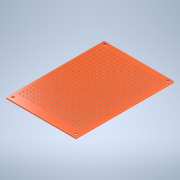
# Autodesk Inventor part: podložka na arduino
Saved by Autodesk Inventor 2022 (Build 260153000, 153)
## iProperties
Created: 2022-02-10
Part Number: podložka na arduino
Material: Generic
Document SubType Name: Modeling
Designer: matys
Density: 1 g/cm^3
Appearance: Smooth - Light Orange
Author: matys
Autodesk Inventor part; units mm, degrees
ref_plane "YZ Plane" through (0, 0, 0) normal (1, 0, 0) x (0, 1, 0)
ref_plane "XZ Plane" through (0, 0, 0) normal (0, 1, 0) x (-1, 0, 0)
ref_plane "XY Plane" through (0, 0, 0) normal (0, 0, 1) x (1, 0, 0)
sketch "Sketch1" plane through (0, 0, 0) normal (0, 1, 0) x (-1, 0, 0)
  line L0 (0, 0) -> (0, -70)
  line L1 (0, -70) -> (50, -70)
  line L2 (50, -70) -> (50, 0)
  line L3 (50, 0) -> (0, 0)
  dimension "d0" = 70
  dimension "d1" = 50
  constraints: 8 end point, 3 perpendicular, 1 vertical
  measures "d0" distance of L0.start L0.end
  measures "d1" distance of L0.end L1.end
extrude "Extrusion1" add sketch "Sketch1" along normal blind 1
sketch "Sketch2" plane through (0, 1, 0) normal (0, 1, 0) x (1, 0, 0)
  line L0 (0, 70) -> (-50, 70) projected
  line L1 (-50, 70) -> (-50, 68)
  line L2 (-50, 70) -> (-50, 0) projected
  line L3 (-50, 68) -> (-47.5, 68)
  line L4 (-47.5, 68) -> (-47.5, 70)
  line L5 (-47.5, 70) -> (-50, 70)
  line L6 (-50, 70) -> (0, 70)
  line L7 (0, 70) -> (-25, 70)
  line L8 (-25, 70) -> (-25, 0)
  line L9 (-25, 0) -> (-25, 70)
  circle A0 centre (-47.5, 68) radius 1
  circle A1 centre (-2.5, 68) radius 1
  line L10 (-50, 0) -> (-50, 2.5)
  line L11 (-50, 2.5) -> (-47.5, 2.5)
  line L12 (-47.5, 2.5) -> (-47.5, 0)
  line L13 (-50, 0) -> (0, 0) projected
  circle A2 centre (-47.5, 2.5) radius 1
  circle A3 centre (-2.5, 2.5) radius 1
  line L14 (-50, 70) -> (-47, 70)
  line L15 (-47, 70) -> (-47, 64.5)
  line L16 (-47, 64.5) -> (-50, 64.5)
  circle A4 centre (-47, 64.5) radius 0.5
  circle A5 centre (-47, 62) radius 0.5
  circle A6 centre (-47, 59.5) radius 0.5
  circle A7 centre (-47, 57) radius 0.5
  circle A8 centre (-47, 54.5) radius 0.5
  circle A9 centre (-47, 52) radius 0.5
  circle A10 centre (-47, 49.5) radius 0.5
  circle A11 centre (-47, 47) radius 0.5
  circle A12 centre (-47, 44.5) radius 0.5
  circle A13 centre (-47, 42) radius 0.5
  circle A14 centre (-47, 39.5) radius 0.5
  circle A15 centre (-47, 37) radius 0.5
  circle A16 centre (-47, 34.5) radius 0.5
  circle A17 centre (-47, 32) radius 0.5
  circle A18 centre (-47, 29.5) radius 0.5
  circle A19 centre (-47, 27) radius 0.5
  circle A20 centre (-47, 24.5) radius 0.5
  circle A21 centre (-47, 22) radius 0.5
  circle A22 centre (-47, 19.5) radius 0.5
  circle A23 centre (-47, 17) radius 0.5
  circle A24 centre (-47, 14.5) radius 0.5
  circle A25 centre (-47, 12) radius 0.5
  circle A26 centre (-47, 9.5) radius 0.5
  circle A27 centre (-47, 7) radius 0.5
  circle A28 centre (-44.5, 64.5) radius 0.5
  circle A29 centre (-44.5, 62) radius 0.5
  circle A30 centre (-44.5, 59.5) radius 0.5
  circle A31 centre (-44.5, 57) radius 0.5
  circle A32 centre (-44.5, 54.5) radius 0.5
  circle A33 centre (-44.5, 52) radius 0.5
  circle A34 centre (-44.5, 49.5) radius 0.5
  circle A35 centre (-44.5, 47) radius 0.5
  circle A36 centre (-44.5, 44.5) radius 0.5
  circle A37 centre (-44.5, 42) radius 0.5
  circle A38 centre (-44.5, 39.5) radius 0.5
  circle A39 centre (-44.5, 37) radius 0.5
  circle A40 centre (-44.5, 34.5) radius 0.5
  circle A41 centre (-44.5, 32) radius 0.5
  circle A42 centre (-44.5, 29.5) radius 0.5
  circle A43 centre (-44.5, 27) radius 0.5
  circle A44 centre (-44.5, 24.5) radius 0.5
  circle A45 centre (-44.5, 22) radius 0.5
  circle A46 centre (-44.5, 19.5) radius 0.5
  circle A47 centre (-44.5, 17) radius 0.5
  circle A48 centre (-44.5, 14.5) radius 0.5
  circle A49 centre (-44.5, 12) radius 0.5
  circle A50 centre (-44.5, 9.5) radius 0.5
  circle A51 centre (-44.5, 7) radius 0.5
  circle A52 centre (-42, 64.5) radius 0.5
  circle A53 centre (-42, 62) radius 0.5
  circle A54 centre (-42, 59.5) radius 0.5
  circle A55 centre (-42, 57) radius 0.5
  circle A56 centre (-42, 54.5) radius 0.5
  circle A57 centre (-42, 52) radius 0.5
  circle A58 centre (-42, 49.5) radius 0.5
  circle A59 centre (-42, 47) radius 0.5
  circle A60 centre (-42, 44.5) radius 0.5
  circle A61 centre (-42, 42) radius 0.5
  circle A62 centre (-42, 39.5) radius 0.5
  circle A63 centre (-42, 37) radius 0.5
  circle A64 centre (-42, 34.5) radius 0.5
  circle A65 centre (-42, 32) radius 0.5
  circle A66 centre (-42, 29.5) radius 0.5
  circle A67 centre (-42, 27) radius 0.5
  circle A68 centre (-42, 24.5) radius 0.5
  circle A69 centre (-42, 22) radius 0.5
  circle A70 centre (-42, 19.5) radius 0.5
  circle A71 centre (-42, 17) radius 0.5
  circle A72 centre (-42, 14.5) radius 0.5
  circle A73 centre (-42, 12) radius 0.5
  circle A74 centre (-42, 9.5) radius 0.5
  circle A75 centre (-42, 7) radius 0.5
  circle A76 centre (-39.5, 64.5) radius 0.5
  circle A77 centre (-39.5, 62) radius 0.5
  circle A78 centre (-39.5, 59.5) radius 0.5
  circle A79 centre (-39.5, 57) radius 0.5
  circle A80 centre (-39.5, 54.5) radius 0.5
  circle A81 centre (-39.5, 52) radius 0.5
  circle A82 centre (-39.5, 49.5) radius 0.5
  circle A83 centre (-39.5, 47) radius 0.5
  circle A84 centre (-39.5, 44.5) radius 0.5
  circle A85 centre (-39.5, 42) radius 0.5
  circle A86 centre (-39.5, 39.5) radius 0.5
  circle A87 centre (-39.5, 37) radius 0.5
  circle A88 centre (-39.5, 34.5) radius 0.5
  circle A89 centre (-39.5, 32) radius 0.5
  circle A90 centre (-39.5, 29.5) radius 0.5
  circle A91 centre (-39.5, 27) radius 0.5
  circle A92 centre (-39.5, 24.5) radius 0.5
  circle A93 centre (-39.5, 22) radius 0.5
  circle A94 centre (-39.5, 19.5) radius 0.5
  circle A95 centre (-39.5, 17) radius 0.5
  circle A96 centre (-39.5, 14.5) radius 0.5
  circle A97 centre (-39.5, 12) radius 0.5
  circle A98 centre (-39.5, 9.5) radius 0.5
  circle A99 centre (-39.5, 7) radius 0.5
  circle A100 centre (-37, 64.5) radius 0.5
  circle A101 centre (-37, 62) radius 0.5
  circle A102 centre (-37, 59.5) radius 0.5
  circle A103 centre (-37, 57) radius 0.5
  circle A104 centre (-37, 54.5) radius 0.5
  circle A105 centre (-37, 52) radius 0.5
  circle A106 centre (-37, 49.5) radius 0.5
  circle A107 centre (-37, 47) radius 0.5
  circle A108 centre (-37, 44.5) radius 0.5
  circle A109 centre (-37, 42) radius 0.5
  circle A110 centre (-37, 39.5) radius 0.5
  circle A111 centre (-37, 37) radius 0.5
  circle A112 centre (-37, 34.5) radius 0.5
  circle A113 centre (-37, 32) radius 0.5
  circle A114 centre (-37, 29.5) radius 0.5
  circle A115 centre (-37, 27) radius 0.5
  circle A116 centre (-37, 24.5) radius 0.5
  circle A117 centre (-37, 22) radius 0.5
  circle A118 centre (-37, 19.5) radius 0.5
  circle A119 centre (-37, 17) radius 0.5
  circle A120 centre (-37, 14.5) radius 0.5
  circle A121 centre (-37, 12) radius 0.5
  circle A122 centre (-37, 9.5) radius 0.5
  circle A123 centre (-37, 7) radius 0.5
  circle A124 centre (-34.5, 64.5) radius 0.5
  circle A125 centre (-34.5, 62) radius 0.5
  circle A126 centre (-34.5, 59.5) radius 0.5
  circle A127 centre (-34.5, 57) radius 0.5
  circle A128 centre (-34.5, 54.5) radius 0.5
  circle A129 centre (-34.5, 52) radius 0.5
  circle A130 centre (-34.5, 49.5) radius 0.5
  circle A131 centre (-34.5, 47) radius 0.5
  circle A132 centre (-34.5, 44.5) radius 0.5
  circle A133 centre (-34.5, 42) radius 0.5
  circle A134 centre (-34.5, 39.5) radius 0.5
  circle A135 centre (-34.5, 37) radius 0.5
  circle A136 centre (-34.5, 34.5) radius 0.5
  circle A137 centre (-34.5, 32) radius 0.5
  circle A138 centre (-34.5, 29.5) radius 0.5
  circle A139 centre (-34.5, 27) radius 0.5
  circle A140 centre (-34.5, 24.5) radius 0.5
  circle A141 centre (-34.5, 22) radius 0.5
  circle A142 centre (-34.5, 19.5) radius 0.5
  circle A143 centre (-34.5, 17) radius 0.5
  circle A144 centre (-34.5, 14.5) radius 0.5
  circle A145 centre (-34.5, 12) radius 0.5
  circle A146 centre (-34.5, 9.5) radius 0.5
  circle A147 centre (-34.5, 7) radius 0.5
  circle A148 centre (-32, 64.5) radius 0.5
  circle A149 centre (-32, 62) radius 0.5
  circle A150 centre (-32, 59.5) radius 0.5
  circle A151 centre (-32, 57) radius 0.5
  circle A152 centre (-32, 54.5) radius 0.5
  circle A153 centre (-32, 52) radius 0.5
  circle A154 centre (-32, 49.5) radius 0.5
  circle A155 centre (-32, 47) radius 0.5
  circle A156 centre (-32, 44.5) radius 0.5
  circle A157 centre (-32, 42) radius 0.5
  circle A158 centre (-32, 39.5) radius 0.5
  circle A159 centre (-32, 37) radius 0.5
  circle A160 centre (-32, 34.5) radius 0.5
  circle A161 centre (-32, 32) radius 0.5
  circle A162 centre (-32, 29.5) radius 0.5
  circle A163 centre (-32, 27) radius 0.5
  circle A164 centre (-32, 24.5) radius 0.5
  circle A165 centre (-32, 22) radius 0.5
  circle A166 centre (-32, 19.5) radius 0.5
  circle A167 centre (-32, 17) radius 0.5
  circle A168 centre (-32, 14.5) radius 0.5
  circle A169 centre (-32, 12) radius 0.5
  circle A170 centre (-32, 9.5) radius 0.5
  circle A171 centre (-32, 7) radius 0.5
  circle A172 centre (-29.5, 64.5) radius 0.5
  circle A173 centre (-29.5, 62) radius 0.5
  circle A174 centre (-29.5, 59.5) radius 0.5
  circle A175 centre (-29.5, 57) radius 0.5
  circle A176 centre (-29.5, 54.5) radius 0.5
  circle A177 centre (-29.5, 52) radius 0.5
  circle A178 centre (-29.5, 49.5) radius 0.5
  circle A179 centre (-29.5, 47) radius 0.5
  circle A180 centre (-29.5, 44.5) radius 0.5
  circle A181 centre (-29.5, 42) radius 0.5
  circle A182 centre (-29.5, 39.5) radius 0.5
  circle A183 centre (-29.5, 37) radius 0.5
  circle A184 centre (-29.5, 34.5) radius 0.5
  circle A185 centre (-29.5, 32) radius 0.5
  circle A186 centre (-29.5, 29.5) radius 0.5
  circle A187 centre (-29.5, 27) radius 0.5
  circle A188 centre (-29.5, 24.5) radius 0.5
  circle A189 centre (-29.5, 22) radius 0.5
  circle A190 centre (-29.5, 19.5) radius 0.5
  circle A191 centre (-29.5, 17) radius 0.5
  circle A192 centre (-29.5, 14.5) radius 0.5
  circle A193 centre (-29.5, 12) radius 0.5
  circle A194 centre (-29.5, 9.5) radius 0.5
  circle A195 centre (-29.5, 7) radius 0.5
  circle A196 centre (-27, 64.5) radius 0.5
  circle A197 centre (-27, 62) radius 0.5
  circle A198 centre (-27, 59.5) radius 0.5
  circle A199 centre (-27, 57) radius 0.5
  circle A200 centre (-27, 54.5) radius 0.5
  circle A201 centre (-27, 52) radius 0.5
  circle A202 centre (-27, 49.5) radius 0.5
  circle A203 centre (-27, 47) radius 0.5
  circle A204 centre (-27, 44.5) radius 0.5
  circle A205 centre (-27, 42) radius 0.5
  circle A206 centre (-27, 39.5) radius 0.5
  circle A207 centre (-27, 37) radius 0.5
  circle A208 centre (-27, 34.5) radius 0.5
  circle A209 centre (-27, 32) radius 0.5
  circle A210 centre (-27, 29.5) radius 0.5
  circle A211 centre (-27, 27) radius 0.5
  circle A212 centre (-27, 24.5) radius 0.5
  circle A213 centre (-27, 22) radius 0.5
  circle A214 centre (-27, 19.5) radius 0.5
  circle A215 centre (-27, 17) radius 0.5
  circle A216 centre (-27, 14.5) radius 0.5
  circle A217 centre (-27, 12) radius 0.5
  circle A218 centre (-27, 9.5) radius 0.5
  circle A219 centre (-27, 7) radius 0.5
  circle A220 centre (-24.5, 64.5) radius 0.5
  circle A221 centre (-24.5, 62) radius 0.5
  circle A222 centre (-24.5, 59.5) radius 0.5
  circle A223 centre (-24.5, 57) radius 0.5
  circle A224 centre (-24.5, 54.5) radius 0.5
  circle A225 centre (-24.5, 52) radius 0.5
  circle A226 centre (-24.5, 49.5) radius 0.5
  circle A227 centre (-24.5, 47) radius 0.5
  circle A228 centre (-24.5, 44.5) radius 0.5
  circle A229 centre (-24.5, 42) radius 0.5
  circle A230 centre (-24.5, 39.5) radius 0.5
  circle A231 centre (-24.5, 37) radius 0.5
  circle A232 centre (-24.5, 34.5) radius 0.5
  circle A233 centre (-24.5, 32) radius 0.5
  circle A234 centre (-24.5, 29.5) radius 0.5
  circle A235 centre (-24.5, 27) radius 0.5
  circle A236 centre (-24.5, 24.5) radius 0.5
  circle A237 centre (-24.5, 22) radius 0.5
  circle A238 centre (-24.5, 19.5) radius 0.5
  circle A239 centre (-24.5, 17) radius 0.5
  circle A240 centre (-24.5, 14.5) radius 0.5
  circle A241 centre (-24.5, 12) radius 0.5
  circle A242 centre (-24.5, 9.5) radius 0.5
  circle A243 centre (-24.5, 7) radius 0.5
  circle A244 centre (-22, 64.5) radius 0.5
  circle A245 centre (-22, 62) radius 0.5
  circle A246 centre (-22, 59.5) radius 0.5
  circle A247 centre (-22, 57) radius 0.5
  circle A248 centre (-22, 54.5) radius 0.5
  circle A249 centre (-22, 52) radius 0.5
  circle A250 centre (-22, 49.5) radius 0.5
  circle A251 centre (-22, 47) radius 0.5
  circle A252 centre (-22, 44.5) radius 0.5
  circle A253 centre (-22, 42) radius 0.5
  circle A254 centre (-22, 39.5) radius 0.5
  circle A255 centre (-22, 37) radius 0.5
  circle A256 centre (-22, 34.5) radius 0.5
  circle A257 centre (-22, 32) radius 0.5
  circle A258 centre (-22, 29.5) radius 0.5
  circle A259 centre (-22, 27) radius 0.5
  circle A260 centre (-22, 24.5) radius 0.5
  circle A261 centre (-22, 22) radius 0.5
  circle A262 centre (-22, 19.5) radius 0.5
  circle A263 centre (-22, 17) radius 0.5
  circle A264 centre (-22, 14.5) radius 0.5
  circle A265 centre (-22, 12) radius 0.5
  circle A266 centre (-22, 9.5) radius 0.5
  circle A267 centre (-22, 7) radius 0.5
  circle A268 centre (-19.5, 64.5) radius 0.5
  circle A269 centre (-19.5, 62) radius 0.5
  circle A270 centre (-19.5, 59.5) radius 0.5
  circle A271 centre (-19.5, 57) radius 0.5
  circle A272 centre (-19.5, 54.5) radius 0.5
  circle A273 centre (-19.5, 52) radius 0.5
  circle A274 centre (-19.5, 49.5) radius 0.5
  circle A275 centre (-19.5, 47) radius 0.5
  circle A276 centre (-19.5, 44.5) radius 0.5
  circle A277 centre (-19.5, 42) radius 0.5
  circle A278 centre (-19.5, 39.5) radius 0.5
  circle A279 centre (-19.5, 37) radius 0.5
  circle A280 centre (-19.5, 34.5) radius 0.5
  circle A281 centre (-19.5, 32) radius 0.5
  circle A282 centre (-19.5, 29.5) radius 0.5
  circle A283 centre (-19.5, 27) radius 0.5
  circle A284 centre (-19.5, 24.5) radius 0.5
  circle A285 centre (-19.5, 22) radius 0.5
  circle A286 centre (-19.5, 19.5) radius 0.5
  circle A287 centre (-19.5, 17) radius 0.5
  circle A288 centre (-19.5, 14.5) radius 0.5
  circle A289 centre (-19.5, 12) radius 0.5
  circle A290 centre (-19.5, 9.5) radius 0.5
  circle A291 centre (-19.5, 7) radius 0.5
  circle A292 centre (-17, 64.5) radius 0.5
  circle A293 centre (-17, 62) radius 0.5
  circle A294 centre (-17, 59.5) radius 0.5
  circle A295 centre (-17, 57) radius 0.5
  circle A296 centre (-17, 54.5) radius 0.5
  circle A297 centre (-17, 52) radius 0.5
  circle A298 centre (-17, 49.5) radius 0.5
  circle A299 centre (-17, 47) radius 0.5
  circle A300 centre (-17, 44.5) radius 0.5
  circle A301 centre (-17, 42) radius 0.5
  circle A302 centre (-17, 39.5) radius 0.5
  circle A303 centre (-17, 37) radius 0.5
  circle A304 centre (-17, 34.5) radius 0.5
  circle A305 centre (-17, 32) radius 0.5
  circle A306 centre (-17, 29.5) radius 0.5
  circle A307 centre (-17, 27) radius 0.5
  circle A308 centre (-17, 24.5) radius 0.5
  circle A309 centre (-17, 22) radius 0.5
  circle A310 centre (-17, 19.5) radius 0.5
  circle A311 centre (-17, 17) radius 0.5
  circle A312 centre (-17, 14.5) radius 0.5
  circle A313 centre (-17, 12) radius 0.5
  circle A314 centre (-17, 9.5) radius 0.5
  circle A315 centre (-17, 7) radius 0.5
  circle A316 centre (-14.5, 64.5) radius 0.5
  circle A317 centre (-14.5, 62) radius 0.5
  circle A318 centre (-14.5, 59.5) radius 0.5
  circle A319 centre (-14.5, 57) radius 0.5
  circle A320 centre (-14.5, 54.5) radius 0.5
  circle A321 centre (-14.5, 52) radius 0.5
  circle A322 centre (-14.5, 49.5) radius 0.5
  circle A323 centre (-14.5, 47) radius 0.5
  circle A324 centre (-14.5, 44.5) radius 0.5
  circle A325 centre (-14.5, 42) radius 0.5
  circle A326 centre (-14.5, 39.5) radius 0.5
  circle A327 centre (-14.5, 37) radius 0.5
  circle A328 centre (-14.5, 34.5) radius 0.5
  circle A329 centre (-14.5, 32) radius 0.5
  circle A330 centre (-14.5, 29.5) radius 0.5
  circle A331 centre (-14.5, 27) radius 0.5
  circle A332 centre (-14.5, 24.5) radius 0.5
  circle A333 centre (-14.5, 22) radius 0.5
  circle A334 centre (-14.5, 19.5) radius 0.5
  circle A335 centre (-14.5, 17) radius 0.5
  circle A336 centre (-14.5, 14.5) radius 0.5
  circle A337 centre (-14.5, 12) radius 0.5
  circle A338 centre (-14.5, 9.5) radius 0.5
  circle A339 centre (-14.5, 7) radius 0.5
  circle A340 centre (-12, 64.5) radius 0.5
  circle A341 centre (-12, 62) radius 0.5
  circle A342 centre (-12, 59.5) radius 0.5
  circle A343 centre (-12, 57) radius 0.5
  circle A344 centre (-12, 54.5) radius 0.5
  circle A345 centre (-12, 52) radius 0.5
  circle A346 centre (-12, 49.5) radius 0.5
  circle A347 centre (-12, 47) radius 0.5
  circle A348 centre (-12, 44.5) radius 0.5
  circle A349 centre (-12, 42) radius 0.5
  circle A350 centre (-12, 39.5) radius 0.5
  circle A351 centre (-12, 37) radius 0.5
  circle A352 centre (-12, 34.5) radius 0.5
  circle A353 centre (-12, 32) radius 0.5
  circle A354 centre (-12, 29.5) radius 0.5
  circle A355 centre (-12, 27) radius 0.5
  circle A356 centre (-12, 24.5) radius 0.5
  circle A357 centre (-12, 22) radius 0.5
  circle A358 centre (-12, 19.5) radius 0.5
  circle A359 centre (-12, 17) radius 0.5
  circle A360 centre (-12, 14.5) radius 0.5
  circle A361 centre (-12, 12) radius 0.5
  circle A362 centre (-12, 9.5) radius 0.5
  circle A363 centre (-12, 7) radius 0.5
  circle A364 centre (-9.5, 64.5) radius 0.5
  circle A365 centre (-9.5, 62) radius 0.5
  circle A366 centre (-9.5, 59.5) radius 0.5
  circle A367 centre (-9.5, 57) radius 0.5
  circle A368 centre (-9.5, 54.5) radius 0.5
  circle A369 centre (-9.5, 52) radius 0.5
  circle A370 centre (-9.5, 49.5) radius 0.5
  circle A371 centre (-9.5, 47) radius 0.5
  circle A372 centre (-9.5, 44.5) radius 0.5
  circle A373 centre (-9.5, 42) radius 0.5
  circle A374 centre (-9.5, 39.5) radius 0.5
  circle A375 centre (-9.5, 37) radius 0.5
  circle A376 centre (-9.5, 34.5) radius 0.5
  circle A377 centre (-9.5, 32) radius 0.5
  circle A378 centre (-9.5, 29.5) radius 0.5
  circle A379 centre (-9.5, 27) radius 0.5
  circle A380 centre (-9.5, 24.5) radius 0.5
  circle A381 centre (-9.5, 22) radius 0.5
  circle A382 centre (-9.5, 19.5) radius 0.5
  circle A383 centre (-9.5, 17) radius 0.5
  circle A384 centre (-9.5, 14.5) radius 0.5
  circle A385 centre (-9.5, 12) radius 0.5
  circle A386 centre (-9.5, 9.5) radius 0.5
  circle A387 centre (-9.5, 7) radius 0.5
  circle A388 centre (-7, 64.5) radius 0.5
  circle A389 centre (-7, 62) radius 0.5
  circle A390 centre (-7, 59.5) radius 0.5
  circle A391 centre (-7, 57) radius 0.5
  circle A392 centre (-7, 54.5) radius 0.5
  circle A393 centre (-7, 52) radius 0.5
  circle A394 centre (-7, 49.5) radius 0.5
  circle A395 centre (-7, 47) radius 0.5
  circle A396 centre (-7, 44.5) radius 0.5
  circle A397 centre (-7, 42) radius 0.5
  circle A398 centre (-7, 39.5) radius 0.5
  circle A399 centre (-7, 37) radius 0.5
  circle A400 centre (-7, 34.5) radius 0.5
  circle A401 centre (-7, 32) radius 0.5
  circle A402 centre (-7, 29.5) radius 0.5
  circle A403 centre (-7, 27) radius 0.5
  circle A404 centre (-7, 24.5) radius 0.5
  circle A405 centre (-7, 22) radius 0.5
  circle A406 centre (-7, 19.5) radius 0.5
  circle A407 centre (-7, 17) radius 0.5
  circle A408 centre (-7, 14.5) radius 0.5
  circle A409 centre (-7, 12) radius 0.5
  circle A410 centre (-7, 9.5) radius 0.5
  circle A411 centre (-7, 7) radius 0.5
  circle A412 centre (-4.5, 64.5) radius 0.5
  circle A413 centre (-4.5, 62) radius 0.5
  circle A414 centre (-4.5, 59.5) radius 0.5
  circle A415 centre (-4.5, 57) radius 0.5
  circle A416 centre (-4.5, 54.5) radius 0.5
  circle A417 centre (-4.5, 52) radius 0.5
  circle A418 centre (-4.5, 49.5) radius 0.5
  circle A419 centre (-4.5, 47) radius 0.5
  circle A420 centre (-4.5, 44.5) radius 0.5
  circle A421 centre (-4.5, 42) radius 0.5
  circle A422 centre (-4.5, 39.5) radius 0.5
  circle A423 centre (-4.5, 37) radius 0.5
  circle A424 centre (-4.5, 34.5) radius 0.5
  circle A425 centre (-4.5, 32) radius 0.5
  circle A426 centre (-4.5, 29.5) radius 0.5
  circle A427 centre (-4.5, 27) radius 0.5
  circle A428 centre (-4.5, 24.5) radius 0.5
  circle A429 centre (-4.5, 22) radius 0.5
  circle A430 centre (-4.5, 19.5) radius 0.5
  circle A431 centre (-4.5, 17) radius 0.5
  circle A432 centre (-4.5, 14.5) radius 0.5
  circle A433 centre (-4.5, 12) radius 0.5
  circle A434 centre (-4.5, 9.5) radius 0.5
  circle A435 centre (-4.5, 7) radius 0.5
  point P0 (-47, 68.866)
  point P1 (-47.5, 64.5)
  point P2 (-47, 65)
  point P3 (-47, 67.134)
  dimension "d4" = 2
  dimension "d5" = 2.5
  dimension "d6" = 2
  dimension "d9" = 2.5
  dimension "d10" = 2.5
  dimension "d11" = 2
  dimension "d12" = 3
  dimension "d13" = 5.5
  dimension "d14" = 1
  dimension "d17" = 2.5
  dimension "d20" = 2.5
  constraints: 436 centre point, 28 end point, 7 perpendicular, 6 point on line, 3 coincident, 2 symmetric about line, 2 vertical, 1 collinear, 1 horizontal, 1 midpoint, 864 other
  measures "d4" distance of L0.end L1.end
  measures "d5" distance of L1.end L3.end
  measures "d6" diameter of A0
  measures "d9" distance of L2.end L10.end
  measures "d10" distance of L10.end L11.end
  measures "d11" diameter of A2
  measures "d12" distance of L0.end L14.end
  measures "d13" distance of L14.end L15.end
  measures "d14" diameter of A4
  measures "d17" distance of A4.centre A5.centre
  measures "d20" distance of A4.centre A28.centre
extrude "Extrusion2" cut sketch "Sketch2" against normal through all contours A220 | A221 | A222 | A223 | A224 | A225 | A226 | A227 | A228 | A229 | A230 | A231 | A232 | A233 | A234 | A235 | A236 | A237 | A238 | A239 | A240 | A241 | A242 | A243 | L15 A0 L3 L4 | A0 L15 | L4 L3 A0 | A4 L16 L15 | L15 L16 A4 | A2 L12 L11 | L11 L12 A2 | A1 | A3 | A5 | A6 | A7 | A8 | A9 | A10 | A11 | A12 | A13 | A14 | A15 | A16 | A17 | A18 | A19 | A20 | A21 | A22 | A23 | A24 | A25 | A26 | A27 | A28 | A29 | A30 | A31 | A32 | A33 | A34 | A35 | A36 | A37 | A38 | A39 | A40 | A41 | A42 | A43 | A44 | A45 | A46 | A47 | A48 | A49 | A50 | A51 | A52 | A53 | A54 | A55 | A56 | A57 | A58 | A59 | A60 | A61 | A62 | A63 | A64 | A65 | A66 | A67 | A68 | A69 | A70 | A71 | A72 | A73 | A74 | A75 | A76 | A77 | A78 | A79 | A80 | A81 | A82 | A83 | A84 | A85 | A86 | A87 | A88 | A89 | A90 | A91 | A92 | A93 | A94 | A95 | A96 | A97 | A98 | A99 | A100 | A101 | A102 | A103 | A104 | A105 | A106 | A107 | A108 | A109 | A110 | A111 | A112 | A113 | A114 | A115 | A116 | A117 | A118 | A119 | A120 | A121 | A122 | A123 | A124 | A125 | A126 | A127 | A128 | A129 | A130 | A131 | A132 | A133 | A134 | A135 | A136 | A137 | A138 | A139 | A140 | A141 | A142 | A143 | A144 | A145 | A146 | A147 | A148 | A149 | A150 | A151 | A152 | A153 | A154 | A155 | A156 | A157 | A158 | A159 | A160 | A161 | A162 | A163 | A164 | A165 | A166 | A167 | A168 | A169 | A170 | A171 | A172 | A173 | A174 | A175 | A176 | A177 | A178 | A179 | A180 | A181 | A182 | A183 | A184 | A185 | A186 | A187 | A188 | A189 | A190 | A191 | A192 | A193 | A194 | A195 | A196 | A197 | A198 | A199 | A200 | A201 | A202 | A203 | A204 | A205 | A206 | A207 | A208 | A209 | A210 | A211 | A212 | A213 | A214 | A215 | A216 | A217 | A218 | A219 | A244 | A245 | A246 | A247 | A248 | A249 | A250 | A251 | A252 | A253 | A254 | A255 | A256 | A257 | A258 | A259 | A260 | A261 | A262 | A263 | A264 | A265 | A266 | A267 | A268 | A269 | A270 | A271 | A272 | A273 | A274 | A275 | A276 | A277 | A278 | A279 | A280 | A281 | A282 | A283 | A284 | A285 | A286 | A287 | A288 | A289 | A290 | A291 | A292 | A293 | A294 | A295 | A296 | A297 | A298 | A299 | A300 | A301 | A302 | A303 | A304 | A305 | A306 | A307 | A308 | A309 | A310 | A311 | A312 | A313 | A314 | A315 | A316 | A317 | A318 | A319 | A320 | A321 | A322 | A323 | A324 | A325 | A326 | A327 | A328 | A329 | A330 | A331 | A332 | A333 | A334 | A335 | A336 | A337 | A338 | A339 | A340 | A341 | A342 | A343 | A344 | A345 | A346 | A347 | A348 | A349 | A350 | A351 | A352 | A353 | A354 | A355 | A356 | A357 | A358 | A359 | A360 | A361 | A362 | A363 | A364 | A365 | A366 | A367 | A368 | A369 | A370 | A371 | A372 | A373 | A374 | A375 | A376 | A377 | A378 | A379 | A380 | A381 | A382 | A383 | A384 | A385 | A386 | A387 | A388 | A389 | A390 | A391 | A392 | A393 | A394 | A395 | A396 | A397 | A398 | A399 | A400 | A401 | A402 | A403 | A404 | A405 | A406 | A407 | A408 | A409 | A410 | A411 | A412 | A413 | A414 | A415 | A416 | A417 | A418 | A419 | A420 | A421 | A422 | A423 | A424 | A425 | A426 | A427 | A428 | A429 | A430 | A431 | A432 | A433 | A434 | A435
body "Solid1"
